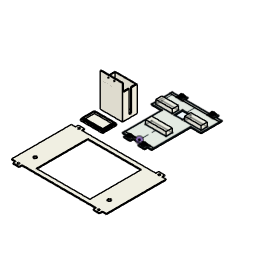
SD Plus Bracket (Autodesk Fusion 360 design; units mm, degrees)
Autodesk Fusion 360 part; units mm, degrees
sketch "Sketch1" plane through (0, 0, 0) normal (0, 0, 1) x (1, 0, 0) in component "SD Plus Back"
  line L0 (-35, 0) -> (35, 0)
  line L1 (60, 90) -> (60, 135)
  line L2 (60, 135) -> (-60, 135)
  line L3 (-60, 135) -> (-60, 90)
  line L4 (-25, 55) -> (25, 55)
  line L5 (25, 55) -> (25, 40)
  line L6 (25, 40) -> (-25, 40)
  line L7 (-25, 40) -> (-25, 55)
  line L8 (0, 0) -> (0, 40) construction
  line L9 (-55, 135) -> (-55, 110) construction
  line L10 (-55, 110) -> (-15, 110)
  line L11 (-15, 110) -> (-15, 95)
  line L12 (-15, 95) -> (-55, 95)
  line L13 (-55, 95) -> (-55, 110)
  line L14 (15, 110) -> (55, 110)
  line L15 (55, 110) -> (55, 95)
  line L16 (55, 95) -> (15, 95)
  line L17 (15, 95) -> (15, 110)
  line L18 (-60, 140) -> (-60, 135)
  line L19 (60, 140) -> (60, 135)
  line L20 (-25, 0) -> (-10, 0)
  line L21 (-10, 0) -> (-10, -12)
  line L22 (-10, -12) -> (-25, -12)
  line L23 (-25, -12) -> (-25, 0)
  line L24 (-17.5, 0) -> (-17.5, -12) construction
  circle A0 centre (-17.5, -6) radius 2.5
  line L25 (-25, -5) -> (-35, -5)
  line L26 (10, 0) -> (25, 0)
  line L27 (25, 0) -> (25, -12)
  line L28 (25, -12) -> (10, -12)
  line L29 (10, -12) -> (10, 0)
  line L30 (17.5, 0) -> (17.5, -12) construction
  circle A1 centre (17.5, -6) radius 2.5
  line L31 (35, -5) -> (25, -5)
  line L32 (10, -5) -> (-10, -5)
  line L33 (-30, 135) -> (-45, 135)
  line L34 (-45, 135) -> (-45, 147)
  line L35 (-45, 147) -> (-30, 147)
  line L36 (-30, 147) -> (-30, 135)
  line L37 (-37.5, 147) -> (-37.5, 135) construction
  circle A2 centre (-37.5, 141) radius 2.5
  line L38 (-60, 140) -> (-45, 140)
  line L39 (30, 135) -> (45, 135)
  line L40 (45, 135) -> (45, 147)
  line L41 (45, 147) -> (30, 147)
  line L42 (30, 147) -> (30, 135)
  line L43 (37.5, 147) -> (37.5, 135) construction
  circle A3 centre (37.5, 141) radius 2.5
  line L44 (-30, 140) -> (30, 140)
  line L45 (45, 140) -> (60, 140)
  line L46 (-35, -5) -> (-35, 90)
  line L47 (-35, 90) -> (-60, 90)
  line L48 (35, -5) -> (35, 90)
  line L49 (35, 90) -> (60, 90)
  line L50 (-10, 115) -> (10, 115)
  line L51 (10, 115) -> (10, 95)
  line L52 (10, 95) -> (-10, 95)
  line L53 (-10, 95) -> (-10, 115)
  line L54 (0, 135) -> (0, 115) construction
  dimension "d5" = 50
  dimension "d6" = 40
  dimension "d7" = 15
  dimension "d8" = 25
  dimension "d10" = 15
  dimension "d11" = 40
  dimension "d17" = 10
  dimension "d18" = 12
  dimension "d19" = 15
  dimension "d20" = 5
  dimension "d21" = 10
  dimension "d23" = 30
  dimension "d24" = 30
  dimension "d27" = 10
  dimension "d29" = 5
  dimension "d30" = 5
  dimension "d31" = 10
  dimension "d33" = 5
  dimension "d34" = 5
  dimension "d35" = 135
  dimension "d36" = 20
  dimension "d37" = 20
  dimension "d38" = 20
  dimension "d39" = 15
  dimension "d40" = 15
  dimension "d41" = 5
  constraint horizontal L0
  constraint vertical L1
  constraint horizontal L2
  constraint vertical L3
  constraint horizontal L4
  constraint vertical L5
  constraint horizontal L6
  constraint vertical L7
  constraint coincident L8.start origin
  constraint midpoint L6 L8.end
  constraint perpendicular L6 L8
  constraint coincident L2 L9.start
  constraint perpendicular L2 L9
  constraint horizontal L10
  constraint vertical L11
  constraint horizontal L12
  constraint vertical L13
  constraint coincident L9.end L10.start
  constraint horizontal L14
  constraint vertical L15
  constraint horizontal L16
  constraint vertical L17
  constraint equal L11 L17
  constraint equal L12 L16
  constraint collinear L10 L14
  constraint horizontal L38
  constraint horizontal L31
  constraint vertical L19
  constraint vertical L18
  constraint horizontal L20
  constraint vertical L21
  constraint horizontal L22
  constraint vertical L23
  constraint coincident L0 L20.start
  constraint midpoint L20 L24.start
  constraint midpoint L22 L24.end
  constraint midpoint L24 A0.centre
  constraint coincident L21 L32.end
  constraint collinear L25 L31
  constraint coincident L23 L25.start
  constraint horizontal L26
  constraint vertical L27
  constraint horizontal L28
  constraint vertical L29
  constraint coincident L0 L26.start
  constraint equal L23 L29
  constraint equal L22 L28
  constraint midpoint L26 L30.start
  constraint midpoint L28 L30.end
  constraint midpoint L30 A1.centre
  constraint equal A0 A1
  constraint coincident L27 L31.end
  constraint collinear L31 L32
  constraint coincident L29 L32.start
  constraint horizontal L33
  constraint vertical L34
  constraint horizontal L35
  constraint vertical L36
  constraint coincident L2 L33.start
  constraint equal L22 L35
  constraint equal L21 L36
  constraint midpoint L35 L37.start
  constraint midpoint L33 L37.end
  constraint midpoint L37 A2.centre
  constraint equal A0 A2
  constraint coincident L36 L44.start
  constraint collinear L38 L44
  constraint coincident L34 L38.end
  constraint horizontal L39
  constraint vertical L40
  constraint horizontal L41
  constraint vertical L42
  constraint coincident L2 L39.start
  constraint equal L22 L41
  constraint equal L23 L40
  constraint midpoint L41 L43.start
  constraint midpoint L39 L43.end
  constraint midpoint L43 A3.centre
  constraint equal A0 A3
  constraint coincident L40 L45.start
  constraint collinear L44 L45
  constraint coincident L42 L44.end
  constraint perpendicular L25 L46
  constraint perpendicular L3 L47
  constraint coincident L46 L0.start
  constraint coincident L8.start L0
  constraint perpendicular L31 L48
  constraint perpendicular L1 L49
  constraint coincident L48 L0.end
  constraint equal L47 L49
  constraint horizontal L50
  constraint vertical L51
  constraint horizontal L52
  constraint vertical L53
  constraint midpoint L2 L54.start
  constraint midpoint L50 L54.end
  constraint perpendicular L50 L54
  measures "d5" distance of L4.start L4.end
  measures "d6" distance of L8.start L8.end
  measures "d7" distance of L4.end L5.end
  measures "d8" distance of L9.start L9.end
  measures "d10" distance of L9.end L12.end
  measures "d11" distance of L11.end L12.end
  measures "d17" distance of L8 L21
  measures "d18" distance of L20.start L22.end
  measures "d19" distance of L21.end L22.end
  measures "d20" diameter of A0
  measures "d21" distance of L8 L29
  measures "d23" distance of L8 L36
  measures "d24" distance of L8.start L42
  measures "d27" distance of L23 L46
  measures "d29" distance of L0 L32
  measures "d30" distance of L2 L44
  measures "d31" distance of L27 L48
  measures "d33" distance of L16 L49
  measures "d34" distance of L12 L47
  measures "d35" distance of L0 L2
  measures "d36" distance of L2 L50
  measures "d37" distance of L50.start L52.end
  measures "d38" distance of L51.end L52.end
  measures "d39" distance of L11 L54
  measures "d40" distance of L17 L54
  measures "d41" distance of L3 L13
extrude "Extrude2" add sketch "Sketch1" against normal blind 2 contours L0 L1 L2 L3 L20 L26 L33 L39 L46 L47 L48 L49 | L0 L23 L25 L46 | L0 L20 L21 L22 L23 | L0 L21 L29 L32 | L0 L26 L27 L28 L29 | L2 L18 L34 L38 | L0 L27 L31 L48 | L2 L33 L34 L35 L36 | L2 L36 L42 L44 | L2 L39 L40 L41 L42 | L2 L19 L40 L45 | L4 L5 L6 L7 | L10 L11 L12 L13 | L14 L15 L16 L17 makes body 1 in component "SD Plus Back"
extrude "Extrude3" add sketch "Sketch1" along normal blind 10 contours L4 L5 L6 L7 | L10 L11 L12 L13 | L14 L15 L16 L17 bodies 1 in component "SD Plus Back"
sketch "Sketch1 (2)" plane through (0, 0, 0) normal (0, 0, 1) x (1, 0, 0) in component "SD Plus Front"
  line L0 (0, 0) -> (0, -50) construction
  line L1 (-70, -55) -> (70, -55) construction
  line L2 (70, -55) -> (70, -190) construction
  line L3 (70, -190) -> (-70, -190) construction
  line L4 (-70, -190) -> (-70, -55) construction
  line L5 (110, -55) -> (110, -190) construction
  line L6 (70, -190) -> (70, -55) construction
  line L7 (-110, -55) -> (-110, -190) construction
  line L8 (-70, -190) -> (-70, -55) construction
  line L9 (-65, -60) -> (65, -60)
  line L10 (65, -60) -> (65, -185)
  line L11 (65, -185) -> (-65, -185)
  line L12 (-65, -185) -> (-65, -60)
  line L13 (115, -50) -> (115, -195)
  line L14 (-115, -195) -> (-115, -50)
  line L15 (-90, -50) -> (-90, -43)
  line L16 (-90, -43) -> (-105, -43)
  line L17 (-105, -43) -> (-105, -50)
  line L18 (-97.5, -43) -> (-97.5, -55) construction
  line L19 (-25, -12) -> (-25, 0) construction
  line L20 (-10, -12) -> (-25, -12) construction
  line L21 (90, -43) -> (105, -43)
  line L22 (105, -43) -> (105, -50)
  line L23 (90, -50) -> (90, -43)
  line L24 (97.5, -43) -> (97.5, -55) construction
  circle A0 centre (-97.5, -49) radius 2.5
  circle A1 centre (-17.5, -6) radius 2.5
  circle A2 centre (97.5, -49) radius 2.5
  line L25 (-115, -50) -> (-105, -50)
  line L26 (-90, -50) -> (90, -50)
  line L27 (105, -50) -> (115, -50)
  line L28 (-90, -195) -> (-90, -202)
  line L29 (-90, -202) -> (-105, -202)
  line L30 (-105, -202) -> (-105, -195)
  line L31 (-97.5, -190) -> (-97.5, -202) construction
  circle A3 centre (-97.5, -196) radius 2.5
  line L32 (-105, -195) -> (-115, -195)
  line L33 (105, -195) -> (105, -202)
  line L34 (105, -202) -> (90, -202)
  line L35 (90, -202) -> (90, -195)
  line L36 (97.5, -190) -> (97.5, -202) construction
  circle A4 centre (97.5, -196) radius 2.5
  line L37 (115, -195) -> (105, -195)
  line L38 (90, -195) -> (-90, -195)
  line L39 (70, -55) -> (110, -55) construction
  line L40 (-70, -55) -> (-110, -55) construction
  line L41 (-110, -190) -> (-70, -190) construction
  line L42 (70, -190) -> (110, -190) construction
  line L43 (90, -190) -> (90, -163) construction
  circle A5 centre (90, -163) radius 4
  circle A6 centre (-90, -163) radius 4
  line L44 (-90, -190) -> (-90, -163) construction
  dimension "d48" = 50
  dimension "d53" = 135
  dimension "d54" = 140
  dimension "d55" = 40
  dimension "d56" = 5
  dimension "d57" = 5
  dimension "d60" = 5
  dimension "d61" = 90
  dimension "d62" = 90
  dimension "d67" = 12
  dimension "d68" = 5
  dimension "d69" = 5
  dimension "d72" = 27
  dimension "d73" = 8
  dimension "d75" = 20
  dimension "d76" = 230
  constraint coincident L0.start origin
  constraint vertical L0
  constraint horizontal L1
  constraint vertical L2
  constraint horizontal L3
  constraint vertical L4
  constraint vertical L5
  constraint vertical L6
  constraint vertical L7
  constraint vertical L8
  constraint coincident L3.end L4.start
  constraint coincident L2.end L3.start
  constraint horizontal L25
  constraint vertical L13
  constraint horizontal L37
  constraint vertical L14
  constraint vertical L15
  constraint horizontal L16
  constraint vertical L17
  constraint midpoint L16 L18.start
  constraint equal L16 L20
  constraint horizontal L21
  constraint vertical L22
  constraint vertical L23
  constraint equal L16 L21
  constraint midpoint L21 L24.start
  constraint midpoint L18 A0.centre
  constraint equal A0 A1
  constraint midpoint L24 A2.centre
  constraint equal A0 A2
  constraint collinear L25 L26
  constraint coincident L0.end L25
  constraint collinear L26 L27
  constraint equal L25 L27
  constraint vertical L28
  constraint horizontal L29
  constraint vertical L30
  constraint equal L16 L29
  constraint collinear L17 L30
  constraint midpoint L29 L31.end
  constraint midpoint L31 A3.centre
  constraint equal A0 A3
  constraint collinear L32 L37
  constraint vertical L33
  constraint horizontal L34
  constraint vertical L35
  constraint equal L29 L34
  constraint collinear L22 L33
  constraint midpoint L34 L36.end
  constraint midpoint L36 A4.centre
  constraint equal A3 A4
  constraint collinear L37 L38
  constraint perpendicular L5 L39
  constraint vertical L24
  constraint perpendicular L7 L40
  constraint equal L39 L40
  constraint vertical L18
  constraint equal L18 L24
  constraint coincident L18.end L40
  constraint coincident L24.end L39
  constraint perpendicular L4 L41
  constraint coincident L31.start L41
  constraint vertical L31
  constraint equal L18 L31
  constraint perpendicular L5 L42
  constraint coincident L36.start L42
  constraint collinear L29 L34
  constraint coincident L42 L43.start
  constraint perpendicular L42 L43
  constraint coincident L43.end A5.centre
  constraint midpoint L42 L43.start
  constraint midpoint L41 L44.start
  constraint perpendicular L41 L44
  constraint equal L43 L44
  constraint coincident A6.centre L44.end
  constraint equal A5 A6
  measures "d48" distance of L0.start L0.end
  measures "d53" distance of L1.start L3.end
  measures "d54" distance of L1.start L1.end
  measures "d55" distance of L1.end L5.start
  measures "d57" distance of L7 L14
  measures "d60" distance of L5 L13
  measures "d61" distance of L0 L15
  measures "d62" distance of L0 L23
  measures "d67" distance of L18.start L18.end
  measures "d68" distance of L26 L40
  measures "d69" distance of L38 L41
  measures "d72" distance of L43.start L43.end
  measures "d73" diameter of A5
  measures "d75" distance of L2 L43
  measures "d76" distance of L13 L14
extrude "Extrude2'" add sketch "Sketch1 (2)" against normal blind 2 separate body contours L13 L14 L15 L16 L17 L21 L22 L23 L25 L26 L27 L28 L29 L30 L32 L33 L34 L35 L37 L38 makes body 2 in component "SD Plus Front"
sketch "Main Case" plane through (0, 0, 0) normal (0, 0, 1) x (1, 0, 0) in component "Arduino Case v2"
  line L0 (-50, 0) -> (-104, 0)
  line L1 (-104, 0) -> (-104, -34)
  line L2 (-104, -34) -> (-50, -34)
  line L3 (-50, -34) -> (-50, 0)
  line L4 (0, 0) -> (-50, 0) construction
  line L5 (-79.5, -21) -> (-74.5, -21)
  line L6 (-74.5, -29) -> (-79.5, -29)
  arc A0 (-79.5, -21) -> (-79.5, -29) centre (-79.5, -25) ccw
  arc A1 (-74.5, -29) -> (-74.5, -21) centre (-74.5, -25) ccw
  line L7 (-83.5, -25) -> (-70.5, -25) construction
  line L8 (-77, -34) -> (-77, -29) construction
  dimension "d95" = 54
  dimension "d96" = 34
  dimension "d106" = 50
  dimension "d116" = 8
  dimension "d119" = 13
  dimension "d93" = 5
  constraint horizontal L0
  constraint vertical L1
  constraint horizontal L2
  constraint vertical L3
  constraint coincident L4.start origin
  constraint perpendicular L3 L4
  constraint equal A0 A1
  constraint tangent L5 A1
  constraint parallel L0 L5
  constraint tangent L6 A0
  constraint parallel L5 L6
  constraint equal L5 L6
  constraint midpoint A0 L7.start
  constraint midpoint A1 L7.end
  constraint tangent L6 A1
  constraint midpoint L2 L8.start
  constraint midpoint L6 L8.end
  constraint vertical L8
  measures "d95" distance of L1.end L2.end
  measures "d96" distance of L0.end L1.end
  measures "d106" distance of L0.start L4.start
  measures "d116" diameter of A0
  measures "d119" horizontal distance of L7.start L7.end
  measures "d93" distance of L8.start L8.end
extrude "Extrude1" add sketch "Main Case" against normal blind 2 separate body contours L0 L1 L2 L3 | L5 L6 A0 A1 makes body 3 in component "Arduino Case v2"
extrude "Extrude2''" add 1 faces at (-68, -22.6667, 0) along direction (0, 0, 1) blind 60 thin wall 2 inside on bodies 3 bodies 3 in component "Arduino Case v2"
sketch "Side Hole" plane through (-104, 0, 0) normal (-1, 0, 0) x (0, -1, 0) in component "Arduino Case v2"
  line L0 (0, 60) -> (0, -2)
  line L1 (0, -2) -> (34, -2)
  line L2 (34, -2) -> (34, 60)
  line L3 (34, 60) -> (0, 60)
  line L4 (17, -2) -> (17, 8) construction
  circle A0 centre (17, 8) radius 2.5
  line L5 (19.5, 8) -> (19.5, 60)
  line L6 (14.5, 8) -> (14.5, 60)
  dimension "d104" = 5
  dimension "d105" = 10
  constraint midpoint L1 L4.start
  constraint perpendicular L1 L4
  constraint coincident L4.end A0.centre
  constraint coincident A0 L5.start
  constraint coincident L3 L5.end
  constraint perpendicular L3 L5
  constraint coincident A0 L6.start
  constraint coincident L3 L6.end
  constraint perpendicular L3 L6
  constraint tangent A0 L6
  constraint tangent A0 L5
  measures "d104" diameter of A0
  measures "d105" distance of L4.start L4.end
extrude "Extrude3'" cut sketch "Side Hole" against normal through all contours L3 A0 L5 L6 | A0 bodies 3 in component "Arduino Case v2"
chamfer "Chamfer1" distance 0.5 angle 45 6 edges at (-77, -34, 60) (-50, -26.75, 60) (-50, -7.25, 60) (-77, 0, 60) (-104, -7.25, 60) (-104, -26.75, 60) on bodies 3 in component "Arduino Case v2"
sketch "Mounting Hole" plane through (0, -34, 0) normal (0, -1, 0) x (1, 0, 0) in component "Arduino Case v2"
  line L0 (-50, 59.5) -> (-104, 59.5)
  line L1 (-104, 59.5) -> (-104, -2)
  line L2 (-104, -2) -> (-50, -2)
  line L3 (-50, -2) -> (-50, 59.5)
  line L4 (-50, -2) -> (-104, -2)
  line L5 (-104, -2) -> (-104, 79.5)
  line L6 (-104, 79.5) -> (-50, 79.5)
  line L7 (-50, 79.5) -> (-50, -2)
  circle A0 centre (-84, 74.5) radius 1.5
  circle A1 centre (-70, 74.5) radius 1.5
  dimension "d80" = 20
  dimension "d81" = 5
  dimension "d82" = 3
  dimension "d84" = 20
  dimension "d86" = 20
  dimension "d88" = 5
  constraint horizontal L4
  constraint vertical L5
  constraint horizontal L6
  constraint vertical L7
  constraint coincident L2.end L3.start
  constraint equal L0 L6
  constraint equal A0 A1
  measures "d80" distance of L0 L6
  measures "d81" distance of L6 A0.centre
  measures "d82" diameter of A0
  measures "d84" distance of L5 A0.centre
  measures "d86" distance of L7 A1.centre
  measures "d88" distance of L6 A1.centre
extrude "Extrude5" cut sketch "Main Case" against normal up to surface (2 mm away) contours L5 L6 A0 A1 bodies 3 in component "Arduino Case v2"
fillet "Fillet1" radius 0.5 12 edges at (-52, -19.5, 34) (-52, -17, 5.5) (-52, -14.5, 34) (-102, -14.5, 34) (-102, -17, 5.5) (-102, -19.5, 34) (-104, -19.5, 33.75) (-104, -17, 5.5) (-104, -14.5, 33.75) (-50, -14.5, 33.75) (-50, -17, 5.5) (-50, -19.5, 33.75) on bodies 3 in component "Arduino Case v2"
sketch "Cover" plane through (0, 0, 0) normal (0, 0, 1) x (1, 0, 0) in component "Arduino Case Cover v1"
  line L0 (-79, -45) -> (-25, -45)
  line L1 (-25, -45) -> (-25, -79)
  line L2 (-25, -79) -> (-79, -79)
  line L3 (-79, -79) -> (-79, -45)
  line L4 (-79, -34) -> (-25, -34)
  line L5 (-79, 0) -> (-79, -34)
  line L6 (0, -45) -> (-25, -45) construction
  line L7 (0, 0) -> (0, -45) construction
  line L8 (0, 0) -> (-25, 0) construction
  line L9 (-27, -77) -> (-77, -77)
  line L10 (-77, -77) -> (-77, -47)
  line L11 (-77, -47) -> (-27, -47)
  line L12 (-27, -47) -> (-27, -77)
  line L13 (-29, -75) -> (-75, -75)
  line L14 (-75, -75) -> (-75, -49)
  line L15 (-75, -49) -> (-29, -49)
  line L16 (-29, -49) -> (-29, -75)
  dimension "d125" = 45
  dimension "d131" = 2
  dimension "d132" = 4
  constraint horizontal L0
  constraint vertical L1
  constraint horizontal L2
  constraint vertical L3
  constraint equal L0 L4
  constraint equal L3 L5
  constraint perpendicular L1 L6
  constraint coincident L0.end L1.start
  constraint coincident L7.start L8.start
  constraint vertical L7
  constraint coincident L6.start L7.end
  constraint equal L6 L8
  measures "d125" distance of L7.start L6.start
extrude "Extrude1'" add sketch "Cover" against normal blind 2 separate body contours L0 L1 L2 L3 | L9 L10 L11 L12 | L13 L14 L15 L16 makes body 4 in component "Arduino Case Cover v1"
extrude "Extrude3''" add sketch "Cover" along normal blind 2 contours L0 L1 L2 L3 | L9 L10 L11 L12 bodies 4 in component "Arduino Case Cover v1"
extrude "Extrude4" add sketch "Cover" along normal blind 4 contours L9 L10 L11 L12 bodies 4 in component "Arduino Case Cover v1"
chamfer "Chamfer1'" distance 0.5 angle 45 4 edges at (-52, -79, 2) (-25, -62, 2) (-79, -62, 2) (-52, -45, 2) on bodies 4 in component "Arduino Case Cover v1"
extrude "Extrude6" add sketch "Mounting Hole" along normal blind 2 bodies 3 in component "Arduino Case v2"
chamfer "Chamfer3" distance 2 angle 45 2 edges at (-85.3985, -34, 75.0424) (-71.3985, -34, 75.0424) measured on face at (-82.6178, -35.3333, 75.0827) measured on face at (-68.6178, -35.3333, 75.0827) on bodies 3 in component "Arduino Case v2"
move_body "Move1" bodies 3 to x (1, 0, 0) y (0, 1, 0) z (0, 0, 1) at (0, 40, 0) in component "Arduino Case v2"
move_body "Move2" bodies 3 to x (1, 0, 0) y (0, 1, 0) z (0, 0, 1) at (25, -35, 0) in component "Arduino Case v2"
component "SD Plus Back" placed x (1, 0, 0) y (0, 1, 0) z (0, 0, 1) at (0, 0, 0)
component "SD Plus Front" placed x (1, 0, 0) y (0, 1, 0) z (0, 0, 1) at (0, 0, 0)
component "Arduino Case v2" placed x (1, 0, 0) y (0, 1, 0) z (0, 0, 1) at (0, 0, 0)
component "Arduino Case Cover v1" placed x (1, 0, 0) y (0, 1, 0) z (0, 0, 1) at (0, 0, 0) in component "Arduino Case v2"
equation "SD_Plus_Width = 140 mm"
equation "SD_Plus_Height = 135 mm"
equation "d10 = d7"
equation "d21 = d17"
equation "d24 = d23"
equation "d30 = d29"
equation "d31 = d27"
equation "d34 = d33"
equation "d35 = SD_Plus_Height"
equation "d40 = d39"
equation "SD_Plus_Depth = 28 mm"
equation "Frame_Depth = 38 mm"
equation "d46 = Frame_Depth - SD_Plus_Depth"
equation "d53 = SD_Plus_Height"
equation "d54 = SD_Plus_Width"
equation "d60 = d57"
equation "d62 = d61"
equation "d68 = d57"
equation "d69 = d57"
equation "d86 = d84"
equation "d88 = d81"
named bodies: "Case"
